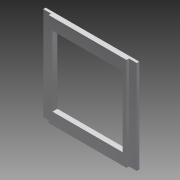
# Autodesk Inventor part: PeltierHeatSinkMount
Saved by Autodesk Inventor 2014 (Build 180170000, 170)
## iProperties
Created: 2015-04-18
Part Number: PeltierHeatSinkMount
Material: Generic
Document SubType Name: Modeling
Designer: Owner
Density: 1 g/cm^3
Appearance: Aluminum - Polished
Author: Owner
Autodesk Inventor part; units mm, degrees
ref_plane "YZ Plane" through (0, 0, 0) normal (1, 0, 0) x (0, 1, 0)
ref_plane "XZ Plane" through (0, 0, 0) normal (0, 1, 0) x (-1, 0, 0)
ref_plane "XY Plane" through (0, 0, 0) normal (0, 0, 1) x (1, 0, 0)
sketch "Sketch1" plane through (0, 0, 0) normal (0, 0, 1) x (1, 0, 0)
  line L0 (-23.4256, 28.8189) -> (21.5744, 28.8189)
  line L1 (21.5744, 28.8189) -> (21.5744, -16.1811)
  line L2 (21.5744, -16.1811) -> (-23.4256, -16.1811)
  line L3 (-23.4256, -16.1811) -> (-23.4256, 28.8189)
  line L4 (-30.9256, 36.3189) -> (29.0744, 36.3189)
  line L5 (29.0744, 36.3189) -> (29.0744, -23.6811)
  line L6 (29.0744, -23.6811) -> (-30.9256, -23.6811)
  line L7 (-30.9256, -23.6811) -> (-30.9256, 36.3189)
  point P0 (0, 0)
  dimension "d0" = 45
  dimension "d1" = 45
  dimension "d2" = 60
  dimension "d3" = 60
  dimension "d4" = 7.5
  dimension "d5" = 7.5
  constraints: 16 end point, 4 parallel, 2 horizontal, 2 perpendicular
  measures "d0" distance of L0.start L0.end
  measures "d1" distance of L0.end L1.end
  measures "d2" distance of L4.start L4.end
  measures "d3" distance of L6.end L4.start
  measures "d4" distance between parallel lines of L3 L7
  measures "d5" distance between parallel lines of L0 L4
extrude "Extrusion1" add sketch "Sketch1" along normal blind 3.175
sketch "Sketch2" plane through (-30.9256, -23.6811, 0) normal (0, -1, 0) x (1, 0, 0)
  line L0 (60, 3.175) -> (55, 3.175)
  line L1 (55, 3.175) -> (55, 1.5875)
  line L2 (55, 1.5875) -> (60, 1.5875)
  line L3 (60, 1.5875) -> (60, 3.175)
  line L4 (0, 3.175) -> (5, 3.175)
  line L5 (5, 3.175) -> (5, 1.5875)
  line L6 (5, 1.5875) -> (0, 1.5875)
  line L7 (0, 1.5875) -> (0, 3.175)
  point P0 (30.9256, 0)
  dimension "d8" = 5
  dimension "d9" = 5
  dimension "d10" = 1.5875
  dimension "d11" = 1.5875
  constraints: 16 end point, 4 parallel, 2 horizontal, 2 perpendicular
  measures "d8" distance of L4.start L4.end
  measures "d9" distance of L1.end L2.end
  measures "d10" distance of L4.end L5.end
  measures "d11" distance of L0.end L1.end
extrude "Extrusion2" cut sketch "Sketch2" against normal through all
sketch "Sketch3" plane through (0, 0, 0) normal (0, 0, -1) x (-1, 0, 0)
  point P0 (-25.0744, 32.3189)
hole "Hole1" at (25.0744, 32.3189, 0) direction (0, 0, 1) diameter 3.4544 depth 1.5875
sketch "Sketch4" plane through (0, 0, 0) normal (0, 0, -1) x (-1, 0, 0)
  point P0 (26.9256, 32.3189)
hole "Hole3" at (-26.9256, 32.3189, 0) direction (0, 0, 1) diameter 3.4544 depth 1.5875
sketch "Sketch5" plane through (0, 0, 0) normal (0, 0, -1) x (-1, 0, 0)
  point P0 (-25.0744, -19.6811)
hole "Hole5" at (25.0744, -19.6811, 0) direction (0, 0, 1) diameter 3.4544 depth 1.5875
sketch "Sketch6" plane through (0, 0, 0) normal (0, 0, -1) x (-1, 0, 0)
  point P0 (26.9256, -19.6811)
hole "Hole7" at (-26.9256, -19.6811, 0) direction (0, 0, 1) diameter 3.4544 depth 1.5875
body "Solid1"
